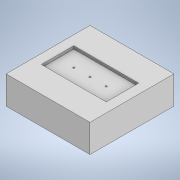
# Autodesk Inventor part: Base_Mount
Saved by Autodesk Inventor 2022 (Build 260153000, 153)
## iProperties
Created: 2022-03-05
Part Number: Base_Mount
Material: Generic
Document SubType Name: Modeling
Designer: Mlees
Density: 1 g/cm^3
Appearance: Default
Author: Mlees
Autodesk Inventor part; units mm, degrees
ref_plane "YZ Plane" through (0, 0, 0) normal (1, 0, 0) x (0, 1, 0)
ref_plane "XZ Plane" through (0, 0, 0) normal (0, 1, 0) x (-1, 0, 0)
ref_plane "XY Plane" through (0, 0, 0) normal (0, 0, 1) x (1, 0, 0)
sketch "Sketch1" plane through (0, 0, 0) normal (0, 1, 0) x (-1, 0, 0)
  line L0 (0, 0) -> (150, 0)
  line L1 (150, 0) -> (150, -150)
  line L2 (150, -150) -> (0, -150)
  line L3 (0, -150) -> (0, 0)
  dimension "d0" = 150
  dimension "d1" = 150
  constraints: 8 end point, 2 parallel, 1 horizontal, 1 perpendicular
  measures "d0" distance of L1.end L2.end
  measures "d1" distance of L0.end L1.end
extrude "Extrusion1" add sketch "Sketch1" along normal blind 50
sketch "Sketch2" plane through (0, 50, 0) normal (0, 1, 0) x (1, 0, 0)
  line L0 (-150, 150) -> (-150, 0) projected
  line L1 (-150, 0) -> (0, 0) projected
  line L2 (-133, 104) -> (-17, 104)
  line L3 (-17, 104) -> (-17, 46)
  line L4 (-17, 46) -> (-133, 46)
  line L5 (-133, 46) -> (-133, 104)
  constraints: 8 end point, 2 parallel, 1 perpendicular
extrude "Extrusion2" cut sketch "Sketch2" against normal blind 5
sketch "Sketch3" plane through (0, 45, 0) normal (0, 1, 0) x (1, 0, 0)
  line L0 (-17, 104) -> (-17, 46) projected
  line L1 (-133, 46) -> (-133, 104) projected
  circle A0 centre (-104, 75) radius 1.5
  circle A1 centre (-75, 75) radius 1.5
  circle A2 centre (-46, 75) radius 1.5
  point P0 (0, 0)
  dimension "d14" = 3
  constraints: 3 centre point
  measures "d14" diameter of A0
extrude "Extrusion3" cut sketch "Sketch3" against normal up to surface (45 mm away)
sketch "Sketch4" plane through (0, 0, 0) normal (0, -1, 0) x (1, 0, 0)
  circle A0 centre (-46, -75) radius 1.5 projected
  circle A1 centre (-46, -75) radius 4
  circle A2 centre (-75, -75) radius 1.5 projected
  circle A3 centre (-75, -75) radius 4
  circle A4 centre (-104, -75) radius 1.5 projected
  circle A5 centre (-104, -75) radius 4
  point P0 (0, 0)
  dimension "d17" = 8
  constraints: 3 centre point, 3 coincident
  measures "d17" diameter of A1
extrude "Extrusion4" cut sketch "Sketch4" against normal blind 25 contours A0 | A1 | A2 | A3 | A4 | A5
body "Solid1"
